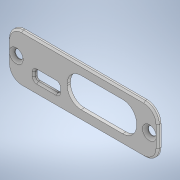
# Autodesk Inventor part: cover
Saved by Autodesk Inventor 2021 (Build 250183000, 183)
## iProperties
Created: 2025-12-12
Part Number: cover
Material: Generic
Document SubType Name: Modeling
Designer: Toby
Density: 1 g/cm^3
Appearance: Default
Author: Toby
Autodesk Inventor part; units mm, degrees
ref_plane "YZ Plane" through (0, 0, 0) normal (1, 0, 0) x (0, 1, 0)
ref_plane "XZ Plane" through (0, 0, 0) normal (0, 1, 0) x (-1, 0, 0)
ref_plane "XY Plane" through (0, 0, 0) normal (0, 0, 1) x (1, 0, 0)
sketch "Sketch1" plane through (0, 0, 0) normal (0, 0, 1) x (1, 0, 0)
  line L0 (-27, 8.75) -> (27, 8.75)
  line L1 (27, 8.75) -> (27, -8.75)
  line L2 (27, -8.75) -> (-27, -8.75)
  line L3 (-27, -8.75) -> (-27, 8.75)
  point P0 (0, 0)
  dimension "d0" = 17.5
  dimension "d1" = 54
  dimension "d2" = 8.75
  dimension "d3" = 27
  constraints: 8 end point, 2 parallel, 1 horizontal, 1 perpendicular
  measures "d0" distance of L2.end L0.start
  measures "d1" distance of L0.start L0.end
  measures "d2" distance from line of point (0, 0) L0
  measures "d3" distance from line of point (0, 0) L3
extrude "Extrusion1" add sketch "Sketch1" along normal blind 1.2
fillet "Fillet1" radius 5 4 edges at (-27, 8.75, 0.6) (-27, -8.75, 0.6) (27, 8.75, 0.6) (27, -8.75, 0.6)
sketch "Sketch2" plane through (0, 0, 1.2) normal (0, 0, 1) x (1, 0, 0)
  line L0 (-22, -8.75) -> (22, -8.75) projected
  line L1 (-27, 3.75) -> (-27, -3.75) projected
  line L2 (27, -3.75) -> (27, 3.75) projected
  point P0 (0, 0)
  point P1 (-24, 0)
  point P2 (24, 0)
  dimension "d7" = 8.75
  dimension "d8" = 8.75
  dimension "d9" = 3
  dimension "d10" = 3
  measures "d7" distance from line of L0 point (-24, 0)
  measures "d8" distance from line of L0 point (24, 0)
  measures "d9" distance from line of L1 point (-24, 0)
  measures "d10" distance from line of L2 point (24, 0)
hole "Hole1" at (-24, 0, 1.2) at (24, 0, 1.2) direction (0, 0, -1) diameter 3 depth 8.8 tip angle 118 countersink diameter 5 countersink angle 90
chamfer "Chamfer1" distance 0.6 angle 45 8 edges at (0, 8.75, 1.2) (-25.5355, 7.2855, 1.2) (-27, 0, 1.2) (-25.5355, -7.2855, 1.2) (0, -8.75, 1.2) (25.5355, -7.2855, 1.2) (27, 0, 1.2) (25.5355, 7.2855, 1.2)
sketch "Sketch3" plane through (0, 0, 1.2) normal (0, 0, 1) x (1, 0, 0)
  line L0 (-21, 6.75) -> (21, 6.75)
  line L1 (21, 6.75) -> (21, -6.75)
  line L2 (21, -6.75) -> (-21, -6.75)
  line L3 (-21, -6.75) -> (-21, 6.75)
  line L4 (22, 8.75) -> (-22, 8.75) projected
  line L5 (-22, -8.75) -> (22, -8.75) projected
  line L6 (-27, 3.75) -> (-27, -3.75) projected
  line L7 (27, -3.75) -> (27, 3.75) projected
  line L8 (-17.6, -1.05) -> (-8.6, -1.05)
  line L9 (-8.6, -1.05) -> (-8.6, -4.55)
  line L10 (-8.6, -4.55) -> (-17.6, -4.55)
  line L11 (-17.6, -4.55) -> (-17.6, -1.05)
  point P0 (0, 0)
  dimension "d21" = 2
  dimension "d22" = 2
  dimension "d23" = 6
  dimension "d24" = 6
  dimension "d25" = 3.4
  dimension "d26" = 9
  dimension "d27" = 3.5
  dimension "d28" = 2.2
  constraints: 16 end point, 4 parallel, 2 horizontal, 2 perpendicular
  measures "d21" distance between parallel lines of L4 L0
  measures "d22" distance between parallel lines of L5 L2
  measures "d23" distance between parallel lines of L6 L3
  measures "d24" distance between parallel lines of L7 L1
  measures "d25" distance between parallel lines of L3 L11
  measures "d26" distance of L8.start L8.end
  measures "d27" distance between parallel lines of L10 L8
  measures "d28" distance between parallel lines of L2 L10
extrude "Extrusion2" cut sketch "Sketch3" against normal blind 1.2 contours L8 L9 L10 L11
sketch "Sketch4" plane through (0, 0, 1.2) normal (0, 0, 1) x (1, 0, 0)
  line L0 (-5.6, 5.55) -> (19.4, 5.55)
  line L1 (19.4, 5.55) -> (19.4, -5.15)
  line L2 (19.4, -5.15) -> (-5.6, -5.15)
  line L3 (-5.6, -5.15) -> (-5.6, 5.55)
  line L4 (22, 8.75) -> (-22, 8.75) projected
  line L5 (-27, 3.75) -> (-27, -3.75) projected
  line L6 (-8.6, -4.55) -> (-17.6, -4.55) projected
  point P0 (0, 0)
  dimension "d31" = 25
  dimension "d32" = 10.7
  dimension "d34" = 21.4
  dimension "d35" = 3.2
  dimension "d36" = 0.6
  constraints: 8 end point, 2 parallel, 1 horizontal, 1 perpendicular
  measures "d31" distance of L0.start L0.end
  measures "d32" distance of L2.end L0.start
  measures "d34" distance between parallel lines of L5 L3
  measures "d35" distance between parallel lines of L4 L0
  measures "d36" distance between parallel lines of L2 L6
extrude "Extrusion3" cut sketch "Sketch4" against normal blind 1.2
fillet "Fillet2" radius 5 4 edges at (-5.6, 5.55, 0.6) (-5.6, -5.15, 0.6) (19.4, 5.55, 0.6) (19.4, -5.15, 0.6)
fillet "Fillet3" radius 1 4 edges at (-8.6, -1.05, 0.6) (-17.6, -1.05, 0.6) (-17.6, -4.55, 0.6) (-8.6, -4.55, 0.6)
sketch "Sketch5" plane through (0, 0, 0) normal (0, 0, -1) x (-1, 0, 0)
  line L0 (8.6, 0.95) -> (17.6, 0.95)
  line L1 (17.6, 0.95) -> (17.6, -1.05)
  line L2 (17.6, -1.05) -> (8.6, -1.05)
  line L3 (8.6, -1.05) -> (8.6, 0.95)
  line L4 (9.6, -1.05) -> (16.6, -1.05) projected
  line L5 (8.6, -3.55) -> (8.6, -2.05) projected
  line L6 (17.6, -2.05) -> (17.6, -3.55) projected
  point P0 (0, 0)
  dimension "d47" = 2
  constraints: 8 end point, 3 collinear, 2 parallel, 1 horizontal, 1 perpendicular
  measures "d47" distance between parallel lines of L2 L0
extrude "Extrusion4" add sketch "Sketch5" along normal blind 4
fillet "Fillet4" radius 1 1 edges at (-13.1, 0.95, 0)
chamfer "Chamfer4" distance 2 angle 45 2 edges at (-8.6, -0.05, -4) (-17.6, -0.05, -4)
chamfer "Chamfer6" distance 0.6 angle 45 8 edges at (-13.1, -1.05, 1.2) (-8.8929, -1.3429, 1.2) (-8.6, -2.8, 1.2) (-8.8929, -4.2571, 1.2) (-13.1, -4.55, 1.2) (-17.3071, -4.2571, 1.2) (-17.6, -2.8, 1.2) (-17.3071, -1.3429, 1.2)
body "Solid1"
